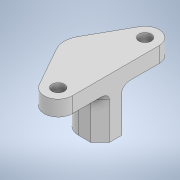
# Autodesk Inventor part: belt_tendor_1
Saved by Autodesk Inventor 2020 (Build 240168000, 168)
## iProperties
Created: 2019-09-03
Part Number: belt_tendor_1
Material: Generic
Document SubType Name: Modeling
Designer: psrob
Density: 1 g/cm^3
Appearance: Default
Author: psrob
Autodesk Inventor part; units mm, degrees
ref_plane "YZ Plane" through (0, 0, 0) normal (1, 0, 0) x (0, 1, 0)
ref_plane "XZ Plane" through (0, 0, 0) normal (0, 1, 0) x (-1, 0, 0)
ref_plane "XY Plane" through (0, 0, 0) normal (0, 0, 1) x (1, 0, 0)
sketch "Sketch1" plane through (0, 0, 0) normal (0, 1, 0) x (-1, 0, 0)
  circle A0 centre (0, 0) radius 2.5
  dimension "d0" = 5
  constraints: 1 centre point, 1 coincident
  measures "d0" diameter of A0
extrude "Extrusion1" add sketch "Sketch1" along normal blind 7
sketch "Sketch2" plane through (0, 7, 0) normal (0, 1, 0) x (1, 0, 0)
  circle A0 centre (0, 0) radius 2.5 projected
  circle A1 centre (0, 0) radius 3.5
  line L0 (0, 0) -> (2.5, 0)
  line L1 (2.5, 0) -> (2.5, 7)
  line L2 (2.5, 0) -> (2.5, -7)
  circle A2 centre (2.5, -7) radius 2.25
  circle A3 centre (2.5, 7) radius 2.25
  line L3 (0, 0) -> (-3.0512, -1.7147)
  line L4 (-3.0512, -1.7147) -> (0.5385, -8.1023)
  line L5 (2.5, -7) -> (0.5385, -8.1023)
  line L6 (2.5, 7) -> (0.5385, 8.1023)
  line L7 (0, 0) -> (-3.0512, 1.7147)
  line L8 (-3.0512, 1.7147) -> (0.5385, 8.1023)
  line L9 (2.5, -7) -> (4.75, -7)
  line L10 (2.5, 7) -> (4.75, 7)
  line L11 (4.75, 7) -> (4.75, -7)
  dimension "d3" = 7
  dimension "d4" = 2.5
  dimension "d5" = 7
  dimension "d6" = 7
  dimension "d7" = 4.5
  dimension "d8" = 4.5
  constraints: 24 end point, 7 point on circle, 5 perpendicular, 3 centre point, 3 coincident, 2 horizontal, 2 vertical, 1 parallel
  measures "d3" diameter of A1
  measures "d4" distance of L0.start L0.end
  measures "d5" distance of L0.end L1.end
  measures "d6" distance of L0.end L2.end
  measures "d7" diameter of A2
  measures "d8" diameter of A3
extrude "Extrusion2" add sketch "Sketch2" along normal blind 3
sketch "Sketch4" plane through (0, 0, 0) normal (0, -1, 0) x (1, 0, 0)
  line L0 (4.75, 7) -> (4.75, -7) projected
  arc A0 (4.75, 7) -> (0.5385, 8.1023) centre (2.5, 7) ccw projected
  line L1 (-3.0512, 1.7147) -> (0.5385, 8.1023) projected
  arc A1 (-3.0512, 1.7147) -> (-3.0512, -1.7147) centre (0, 0) ccw projected
  line L2 (0.5385, -8.1023) -> (-3.0512, -1.7147) projected
  arc A2 (0.5385, -8.1023) -> (4.75, -7) centre (2.5, -7) ccw projected
  circle A3 centre (0, 0) radius 2.5 projected
extrude "Extrusion4" add sketch "Sketch4" along normal blind 3 contours L0 A2 L2 A1 L1 A0 | A3
sketch "Sketch5" plane through (0, 7, 0) normal (0, -1, 0) x (1, 0, 0)
  circle A0 centre (0, 0) radius 2.5 projected
  line L0 (4.75, -7) -> (4.75, 7) projected
  line L1 (0, 0) -> (0, 2.5)
  circle A1 centre (0, 0) radius 2.5 projected
  line L2 (4.75, -7) -> (4.75, 7) projected
  line L3 (0, 2.5) -> (4.75, 2.5)
  line L4 (4.75, 2.5) -> (4.75, -2.5)
  line L5 (4.75, -2.5) -> (0, -2.5)
  line L6 (0, -2.5) -> (0, 2.5)
  point P0 (6.25, 2.5)
  point P1 (4.75, 7.3386)
  point P2 (4.75, 2.5)
  constraints: 10 end point, 2 parallel, 1 horizontal, 1 perpendicular, 1 point on line, 1 vertical, 1 vertical alignment, 1 other
extrude "Extrusion5" add sketch "Sketch5" along normal up to surface (7 mm away) contours A0 L3 L0 L5
sketch "Sketch7" plane through (0, -3, 0) normal (0, -1, 0) x (1, 0, 0)
  arc A0 (0.5385, -8.1023) -> (4.75, -7) centre (2.5, -7) ccw projected
  line L0 (4.75, -7) -> (4.75, 7) projected
  arc A1 (4.75, 7) -> (0.5385, 8.1023) centre (2.5, 7) ccw projected
  line L1 (0.5385, 8.1023) -> (-3.0512, 1.7147) projected
  arc A2 (-3.0512, 1.7147) -> (-3.0512, -1.7147) centre (0, 0) ccw projected
  line L2 (-3.0512, -1.7147) -> (0.5385, -8.1023) projected
  circle A3 centre (2.5, -7) radius 1
  circle A4 centre (2.5, 7) radius 1
  dimension "d27" = 2
  dimension "d28" = 2
  constraints: 2 centre point, 2 coincident
  measures "d27" diameter of A3
  measures "d28" diameter of A4
extrude "Extrusion7" cut sketch "Sketch7" against normal up to surface (13 mm away) contours A3 | A4
thicken "Thicken1" operation add thickness 0.5 both sides no extend neighbours yes toward (0, 1, 0) faces at (0.73, -3, -0.5716)
thicken "Thicken2" operation add thickness 0.5 both sides no extend neighbours yes toward (0, -1, 0) faces at (0.73, 10, 0.5716)
sketch "Sketch8" plane through (0, 0, 0) normal (0, 1, 0) x (1, 0, 0)
  arc A0 (0, 2.5) -> (0, -2.5) centre (0, 0) ccw projected
  line L0 (0, 0) -> (1.5, 0)
  circle A1 centre (1.5, 0) radius 2.5
  line L1 (0, 2.5) -> (4.75, 2.5) projected
  line L2 (4.75, -2.5) -> (0, -2.5) projected
  line L3 (1.5, 0) -> (1.5, 2.5)
  line L4 (1.5, 2.5) -> (0, 2.5)
  line L5 (1.5, 0) -> (1.375, -2.5)
  line L6 (1.375, -2.5) -> (0, -2.5)
  line L7 (0, -2.5) -> (1.5, -2.5)
  line L8 (1.5, -2.5) -> (1.5, 2.5)
  line L9 (1.5, 2.5) -> (0, 2.5)
  line L10 (0, 2.5) -> (0, -2.5)
  point P0 (2.75, 2.5)
  point P1 (2.75, -2.5)
  point P2 (1.3752, -2.4969)
  point P3 (3.75, 2.5)
  point P4 (3.75, -2.5)
  dimension "d36" = 5
  dimension "d35" = 1.5
  constraints: 18 end point, 2 collinear, 2 horizontal, 2 parallel, 2 point on line, 1 coincident, 1 perpendicular, 1 tangent, 3 other
  measures "d35" distance of L0.start L0.end
extrude "Extrusion8" cut sketch "Sketch8" along normal up to surface (7 mm away) contours L10 A1 A0 | L1 A1 L10 | L10 A1 L5 L2
sketch "Sketch11" plane through (0, 7, 0) normal (0, -1, 0) x (1, 0, 0)
  circle A0 centre (2.5, 7) radius 1 projected
  circle A1 centre (2.5, -7) radius 1 projected
  line L0 (-3.0512, 1.7147) -> (0.5385, 8.1023) projected
  arc A2 (4.75, 7) -> (0.5385, 8.1023) centre (2.5, 7) ccw projected
  line L1 (4.75, 7) -> (4.75, -7) projected
  arc A3 (0.5385, -8.1023) -> (4.75, -7) centre (2.5, -7) ccw projected
  line L2 (0.5385, -8.1023) -> (-3.0512, -1.7147) projected
  arc A4 (-3.0512, 1.7147) -> (-3.0512, -1.7147) centre (0, 0) ccw projected
extrude "Extrusion9" cut sketch "Sketch11" along normal up to surface (7 mm away)
sketch "Sketch12" plane through (0, 0, 0) normal (0, 1, 0) x (1, 0, 0)
  circle A0 centre (2.5, -7) radius 1 projected
  circle A1 centre (2.5, 7) radius 1 projected
  line L0 (4.75, 7) -> (4.75, -7) projected
  arc A2 (4.75, 7) -> (0.5385, 8.1023) centre (2.5, 7) ccw projected
  line L1 (-3.0512, 1.7147) -> (0.5385, 8.1023) projected
  arc A3 (-3.0512, 1.7147) -> (-3.0512, -1.7147) centre (0, 0) ccw projected
  line L2 (0.5385, -8.1023) -> (-3.0512, -1.7147) projected
  arc A4 (0.5385, -8.1023) -> (4.75, -7) centre (2.5, -7) ccw projected
  line L3 (4.75, 7) -> (4.75, -7) projected
  line L4 (4.75, 0) -> (3.75, 0)
  line L5 (3.75, 0) -> (1.25, 0)
  circle A5 centre (1.25, 0) radius 2.5
  line L6 (1.25, 0) -> (1.25, -2.5)
  line L7 (1.25, -2.5) -> (4.75, -2.5)
  line L8 (4.75, -2.5) -> (4.75, 2.5)
  line L9 (4.75, 2.5) -> (1.25, 2.5)
  line L10 (1.25, 2.5) -> (1.25, -2.5)
  point P0 (4.75, 2.5)
  dimension "d45" = 1
  dimension "d46" = 2.5
  dimension "d47" = 5
  dimension "d48" = 3.5
  dimension "d49" = 5
  constraints: 14 end point, 3 horizontal, 2 parallel, 2 point on circle, 1 centre point, 1 coincident, 1 midpoint, 1 perpendicular
  measures "d45" distance of L4.start L4.end
  measures "d46" distance of L4.end L5.end
  measures "d47" diameter of A5
  measures "d48" distance of L9.end L8.end
  measures "d49" distance of L8.end L7.end
extrude "Extrusion10" add sketch "Sketch12" along normal up to surface (7 mm away) contours L0 L4 A5 L9 | L0 L7 A5 L4 | L10 L6 A5 | A5 L5 L10 | A5 L6 L5
chamfer "Chamfer2" distance 1.5 angle 45 2 edges at (4.75, 3.5, 2.5) (4.75, 3.5, -2.5)
sketch "Sketch13" plane through (0, 0, 0) normal (0, 1, 0) x (1, 0, 0)
  circle A0 centre (2.5, -7) radius 1 projected
  circle A1 centre (2.5, 7) radius 1 projected
  line L0 (-3.0512, 1.7147) -> (0.5385, 8.1023) projected
  arc A2 (4.75, 7) -> (0.5385, 8.1023) centre (2.5, 7) ccw projected
  line L1 (4.75, 7) -> (4.75, -7) projected
  arc A3 (0.5385, -8.1023) -> (4.75, -7) centre (2.5, -7) ccw projected
  line L2 (0.5385, -8.1023) -> (-3.0512, -1.7147) projected
  arc A4 (-3.0512, 1.7147) -> (-3.0512, -1.7147) centre (0, 0) ccw projected
extrude "Extrusion11" cut sketch "Sketch13" against normal blind 10
sketch "Sketch14" plane through (0, 0, 0) normal (0, -1, 0) x (1, 0, 0)
  line L0 (4.75, -1) -> (3.25, -2.5) projected
  line L1 (4.75, 1) -> (4.75, -1) projected
  line L2 (3.25, 2.5) -> (4.75, 1) projected
  line L3 (3.25, 2.5) -> (1.25, 2.5) projected
  arc A0 (1.25, 2.5) -> (1.25, -2.5) centre (1.25, 0) ccw projected
  line L4 (1.25, -2.5) -> (3.25, -2.5) projected
  circle A1 centre (1.25, 0) radius 1
  point P0 (0, 0)
  dimension "d58" = 2
  constraints: 1 centre point, 1 coincident
  measures "d58" diameter of A1
extrude "Extrusion12" cut sketch "Sketch14" against normal blind 5 contours A1
fillet "Fillet3" radius 1 2 edges at (4, 7, -1.75) (4, 7, 1.75)
body "Solid1"
